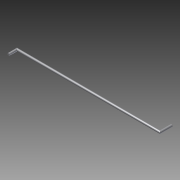
# Autodesk Inventor part: TableMount-ServoWire
Saved by Autodesk Inventor 2012 (Build 160160000, 160)
## iProperties
Created: 2013-07-16
Part Number: TableMount-ServoWire
Material: Default
Document SubType Name: Modeling
Designer: joe_000
Density: 1 g/cm^3
Mass: 0.056855 g
Surface Area: 2.28991 cm^2
Volume: 0.056855 cm^3
Author: joe_000
Autodesk Inventor part; units mm, degrees
ref_plane "YZ Plane" through (0, 0, 0) normal (1, 0, 0) x (0, 1, 0)
ref_plane "XZ Plane" through (0, 0, 0) normal (0, 1, 0) x (-1, 0, 0)
ref_plane "XY Plane" through (0, 0, 0) normal (0, 0, 1) x (1, 0, 0)
sketch "Sketch5" plane through (0, 0, 0) normal (0, 1, 0) x (-1, 0, 0)
  line L0 (0, 0) -> (0, 5.08)
  line L1 (0, 5.08) -> (63.5, 5.08)
  line L2 (63.5, 5.08) -> (63.5, 8.89)
  dimension "d8" = 5.08
  dimension "d9" = 63.5
  dimension "d10" = 3.81
  constraints: 6 end point, 1 coincident, 1 horizontal, 1 parallel, 1 vertical
  measures "d8" distance of L0.start L0.end
  measures "d9" distance of L0.end L1.end
  measures "d10" distance of L1.end L2.end
sketch "Sketch7" plane through (0, 0, 0) normal (0, 0, 1) x (1, 0, 0)
  circle A0 centre (0, 0) radius 0.5
  dimension "WireDiameter" = 1
  constraints: 1 centre point, 1 coincident
  measures "WireDiameter" diameter of A0
sweep "Sweep2" add profiles "Sketch7" path "Sketch5"
body "Solid3"
